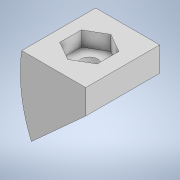
# Autodesk Inventor part: Soporte placa
Saved by Autodesk Inventor 2021 (Build 250183000, 183)
## iProperties
Created: 2020-11-18
Part Number: Soporte placa
Material: Generic
Document SubType Name: Modeling
Designer: Miguel
Density: 1 g/cm^3
Appearance: Default
Author: Miguel
Autodesk Inventor part; units mm, degrees
ref_plane "YZ Plane" through (0, 0, 0) normal (1, 0, 0) x (0, 1, 0)
ref_plane "XZ Plane" through (0, 0, 0) normal (0, 1, 0) x (-1, 0, 0)
ref_plane "XY Plane" through (0, 0, 0) normal (0, 0, 1) x (1, 0, 0)
sketch "Sketch1" plane through (0, 0, 0) normal (0, 0, 1) x (1, 0, 0)
  circle A0 centre (0, 0) radius 28
  line L0 (-27.5, 5.5) -> (27.5, 5.5)
  line L1 (27.5, 5.5) -> (27.5, 4)
  line L2 (27.5, 4) -> (-27.5, 4)
  line L3 (-27.5, 4) -> (-27.5, 5.5)
  line L4 (-27.7128, 4) -> (27.7128, 4)
  line L5 (-14.7128, 4) -> (-14.7128, -1)
  line L6 (-14.7128, -1) -> (-25.7488, -11)
  line L7 (-27.5, 4.75) -> (-21.5, 4.75)
  dimension "d0" = 56
  dimension "d1" = 55
  dimension "d2" = 1.5
  dimension "d3" = 27.5
  dimension "d4" = 4
  dimension "d5" = 4
  dimension "d6" = 5
  dimension "d7" = 13
  dimension "d8" = 15
  dimension "d12" = 6
  dimension "d13" = 6.2128
  constraints: 16 end point, 3 horizontal, 3 point on circle, 2 parallel, 2 perpendicular, 1 centre point, 1 coincident, 1 midpoint, 1 point on line
  measures "d0" diameter of A0
  measures "d1" distance between parallel lines of L1 L3
  measures "d2" distance between parallel lines of L0 L2
  measures "d3" distance from line of point (0, 0) L3
  measures "d4" distance from line of L2 point (0, 0)
  measures "d5" distance from line of point (0, 0) L4
  measures "d6" distance of L5.start L5.end
  measures "d7" distance from line of L4.start L5
  measures "d8" distance from line of L2 L6.end
  measures "d12" distance from line of L3 L7.end
  measures "d13" horizontal distance of L7.end L4.start
extrude "Extrusion1" add sketch "Sketch1" along normal mid plane 15 contours A0 L4 L2 L5 L6 picked at (-22.5928, -6.0493)
sketch "Sketch2" plane through (-27.7128, 4, 7.5) normal (0, 1, 0) x (1, 0, 0)
  line L0 (6.213, 11.8879) -> (10.013, 9.6939)
  line L1 (10.013, 9.6939) -> (10.013, 5.3061)
  line L2 (10.013, 5.3061) -> (6.213, 3.1121)
  line L3 (6.213, 3.1121) -> (2.413, 5.3061)
  line L4 (2.413, 5.3061) -> (2.413, 9.6939)
  line L5 (2.413, 9.6939) -> (6.213, 11.8879)
  line L6 (0, 15) -> (0, 0) projected
  line L7 (13, 15) -> (13, 0) projected
  line L8 (13, 7.5) -> (0, 7.5)
  point P0 (27.7128, 7.5)
  point P1 (6.213, 7.5)
  dimension "d14" = 6.213
  dimension "d15" = 0
  dimension "d16" = 7.6
  constraints: 14 end point, 2 midpoint, 1 parallel, 13 other
  measures "d14" distance from line of L6 point (6.213, 7.5)
  measures "d15" distance from line of L8 point (6.213, 7.5)
  measures "d16" distance between parallel lines of L2 L5
extrude "Extrusion2" cut sketch "Sketch2" against normal blind 3
sketch "Sketch3" plane through (-27.7128, 1, 7.5) normal (0, 1, 0) x (1, 0, 0)
  circle A0 centre (6.213, 7.5) radius 1.75
  point P0 (27.7128, 7.5)
  dimension "d19" = 3.5
  constraints: 1 centre point
  measures "d19" diameter of A0
extrude "Extrusion3" cut sketch "Sketch3" against normal blind 10
body "Solid1"
